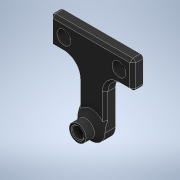
# Autodesk Inventor part: RodHolder_2
Saved by Autodesk Inventor 2021 (Build 250183000, 183)
## iProperties
Created: 2020-07-16
Part Number: RodHolder_2
Material: Generic
Document SubType Name: Modeling
Designer: CASE-SMALL2
Density: 1 g/cm^3
Appearance: Default
Author: CASE-SMALL2
Autodesk Inventor part; units mm, degrees
ref_plane "YZ Plane" through (0, 0, 0) normal (1, 0, 0) x (0, 1, 0)
ref_plane "XZ Plane" through (0, 0, 0) normal (0, 1, 0) x (-1, 0, 0)
ref_plane "XY Plane" through (0, 0, 0) normal (0, 0, 1) x (1, 0, 0)
sketch "Sketch1" plane through (0, 0, 0) normal (0, 0, 1) x (1, 0, 0)
  line L0 (-42, 0) -> (42, 0) projected
  line L1 (-30, 0) -> (-30, -20)
  line L2 (-30, -20) -> (-10, -20)
  line L3 (-10, -20) -> (-10, -65)
  line L4 (-10, -65) -> (0, -65)
  line L5 (0, -78) -> (0, 13) projected
  line L6 (-30, 0) -> (0, 0)
  line L7 (30, 0) -> (30, -20)
  line L8 (30, -20) -> (10, -20)
  line L9 (10, -20) -> (10, -65)
  line L10 (10, -65) -> (0, -65)
  line L11 (30, 0) -> (0, 0)
  line L12 (-30, -10) -> (30, -10) construction
  circle A0 centre (-20, -10) radius 2.4
  circle A1 centre (20, -10) radius 2.4
  dimension "d0" = 10
  dimension "d1" = 20
  dimension "d2" = 65
  dimension "d3" = 30
  dimension "d4" = 10
  dimension "d5" = 4.8
  dimension "d6" = 4.8
  dimension "d7" = 10
  dimension "d8" = 10
  constraints: 22 end point, 4 perpendicular, 4 point on line, 4 symmetric about line, 2 centre point, 2 midpoint, 1 collinear, 1 vertical
  measures "d0" distance from line of L6.end L3
  measures "d1" distance between parallel lines of L0 L2
  measures "d2" distance between parallel lines of L0 L4
  measures "d3" distance between parallel lines of L5 L1
  measures "d4" distance between parallel lines of L11 L12
  measures "d5" diameter of A1
  measures "d6" diameter of A0
  measures "d7" distance from line of L1 A0.centre
  measures "d8" distance from line of L7 A1.centre
extrude "Extrusion1" add sketch "Sketch1" along normal blind 8
sketch "Sketch2" plane through (0, 0, 8) normal (0, 0, 1) x (1, 0, 0)
  circle A0 centre (-20, -10) radius 2.4 projected
  circle A1 centre (20, -10) radius 2.4 projected
  circle A2 centre (-20, -10) radius 5
  circle A3 centre (20, -10) radius 5
  point P0 (0, 0)
  dimension "d11" = 10
  dimension "d12" = 10
  constraints: 2 centre point, 2 coincident
  measures "d11" diameter of A2
  measures "d12" diameter of A3
extrude "Extrusion2" cut sketch "Sketch2" against normal blind 6
sketch "Sketch3" plane through (0, 0, 8) normal (0, 0, 1) x (1, 0, 0)
  line L0 (0, -78) -> (0, 13) projected
  circle A0 centre (0, -55) radius 4.15
  circle A1 centre (-20, -10) radius 2.4 projected
  circle A2 centre (0, -55) radius 6.15
  point P0 (0, 0)
  dimension "d15" = 45
  dimension "d16" = 8.3
  dimension "d17" = 2
  constraints: 2 centre point, 1 coincident, 1 point on line
  measures "d15" vertical distance of A0.centre A1.centre
  measures "d16" diameter of A0
  measures "d17" radial gap between concentric circles of A0 A2
extrude "Extrusion3" add sketch "Sketch3" along normal blind 10 contours A2 L0 A0 | L0 A0 A2
chamfer "Chamfer1" distance 0.5 angle 45 1 edges at (-4.15, -55, 18)
chamfer "Chamfer2" distance 4 angle 45 1 edges at (-6.15, -55, 8)
fillet "Fillet1" radius 10 4 edges at (10, -65, 4) (-10, -65, 4) (-10, -20, 4) (10, -20, 4)
fillet "Fillet2" radius 2 4 edges at (30, -20, 4) (30, 0, 4) (-30, 0, 4) (-30, -20, 4)
chamfer "Chamfer3" distance 0.5 angle 45 9 edges at (-7.0711, -62.0711, 0) (-10, -42.5, 0) (7.0711, -62.0711, 0) (10, -42.5, 0) (23.9999, -20, 0) (-23.9999, -20, 0) (-30, -10, 0) (0, 0, 0) (30, -10, 0)
chamfer "Chamfer4" distance 2 angle 45 9 edges at (-12.9289, -22.9289, 8) (-23.9999, -20, 8) (-10, -41.6307, 8) (-30, -10, 8) (0, 0, 8) (10, -41.6307, 8) (12.9289, -22.9289, 8) (23.9999, -20, 8) (30, -10, 8)
equation "\"d4\" = 0.5 * d1"
equation "\"d8\" = d7"
equation "\"d12\" = d11"
body "Solid1"
